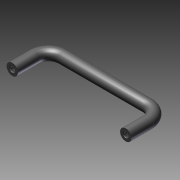
# Autodesk Inventor part: UWANGF_pull100-5
Saved by Autodesk Inventor 2015 SP1 (Build 190203100, 203)
## iProperties
Category: Hardware
Company: MISUMI
Created: 2015-01-28
Part Number: UWANGF_pull100-5
Catalog Web Link: http://us.misumi-ec.com/vona2/detail/110302025920/
Description: UWANGF, UWANSGF_pull-Pulls with Plates - Pull
Vendor: MISUMI
Document SubType Name: Modeling
Designer: psAdmin
Manufacturer: MISUMI
Mass: 11.5881 g
Surface Area: 53.4638 cm^2
Volume: 11.5881 cm^3
Density: 1 g/cm^3
Material: Generic
Appearance: PSOLRGB-192-192-192
Stock Number: UWANGF-100-5
PSOL_IDENT_0: {\\10.0.0.236\data_v8\23d-libs\misumi\metric\39_accessories_for_al_extrusions\uwangf_pull.prj},196 {
PSOL_IDENT_1: VTYP=3D},{NB=UWANGF_pull100-5},{LINA=UWANGF_pull100-5},{NN=UWANGF, UWANSGF_pull},{DATE=17.11.2014 05
PSOL_IDENT_2: :31:37},{GEOMDATE=14.09.2009 00:00:00},{VERSION=},{LINEID=20},{LINESUBID=-1},{WBVAR=MATMB,AF}  {NB=U
PSOL_IDENT_3: WANGF_pull100-5},{LINA=UWANGF_pull100-5},{KT=DUMMY},{PN=UWANGF_pull100-5},{TYPE=UWANGF_pull},{MATMB=
PSOL_IDENT_4: },{STMB=Chrome Plating},{MATP=Zinc Die Cast},{STP=Electrostatic Coating (Siliver)},{MATB=316 Stainle
PSOL_IDENT_5: ss Steel or Equivalent},{MATN=304 Stainless Steel or Equivalent},{MATT=304 Stainless Steel equivalen
PSOL_IDENT_6: t},{L=100},{AF=5},{AF1=5},{P=124},{L1=138},{ND=5},{NC=10.5},{LOAD=2000},{BOLT=SHFBS},{BOLTQ=4},{NUT=
PSOL_IDENT_7: HNTTSN},{NUTQ=2}
SUPPLIER: MISUMI
ARTICLENO: UWANGF_pull100-5
BOMINFO: UWANGF_pull100-5
CREATOR: CADENAS GmbH
Title: Handle
Author: Misumi
Autodesk Inventor part; units mm, degrees
sketch "Sketch_1" plane through (0, 0, 0) normal (0, 1, 0) x (-1, 0, 0)
  circle A0 centre (50, 0) radius 5
  constraints: 1 centre point
extrude "Extrusion1" add sketch "Sketch_1" along normal blind 19
sketch "Sketch_2" plane through (0, 19, 0) normal (0, 1, 0) x (1, 0, 0)
  line L0 (-37, 5) -> (-37, -5)
  circle A0 centre (-50, 0) radius 5
  constraints: 2 end point, 1 centre point
revolve "Revolution1" add sketch "Sketch_2" angle 90 about axis through (-37, 19, -5) along (0, 0, -1)
sketch "Sketch_3" plane through (-37, 0, 0) normal (1, 0, 0) x (0, 0, -1)
  circle A0 centre (0, 32) radius 5
  constraints: 1 centre point
extrude "Extrusion2" add sketch "Sketch_3" along normal blind 74
sketch "Sketch_4" plane through (0, 19, 0) normal (0, 1, 0) x (1, 0, 0)
  line L0 (37, -5) -> (37, 5)
  circle A0 centre (50, 0) radius 5
  constraints: 2 end point, 1 centre point
revolve "Revolution2" add sketch "Sketch_4" angle 90 about axis through (37, 19, 5) along (0, 0, 1)
sketch "Sketch_5" plane through (0, 0, 0) normal (0, 1, 0) x (-1, 0, 0)
  circle A0 centre (-50, 0) radius 5
  constraints: 1 centre point
extrude "Extrusion3" add sketch "Sketch_5" along normal blind 19
sketch "Sketch_6" plane through (0, 0, 0) normal (0, 0, 1) x (1, 0, 0)
  line L0 (-50, 0) -> (-50, 16.1934)
  line L1 (-50, 16.1934) -> (-47.933, 15)
  line L2 (-47.933, 15) -> (-47.933, 0.433)
  line L3 (-47.933, 0.433) -> (-47.5, 0)
  line L4 (-47.5, 0) -> (-50, 0)
  line L5 (-50, 0) -> (-50, 16.1934)
  constraints: 12 end point
revolve "Revolution3" cut sketch "Sketch_6" angle 360 about axis through (-50, 0, 0) along (0, -1, 0)
thread "Thread1" size "M5x0.8" class "6H" standard "ISO Metric profile" length 13 offset 2
sketch "Sketch_7" plane through (0, 0, 0) normal (0, 0, 1) x (1, 0, 0)
  line L0 (50, 0) -> (50, 16.1934)
  line L1 (50, 16.1934) -> (52.067, 15)
  line L2 (52.067, 15) -> (52.067, 0.433)
  line L3 (52.067, 0.433) -> (52.5, 0)
  line L4 (52.5, 0) -> (50, 0)
  line L5 (50, 0) -> (50, 16.1934)
  constraints: 12 end point
revolve "Revolution4" cut sketch "Sketch_7" angle 360 about axis through (50, 0, 0) along (0, -1, 0)
thread "Thread2" size "M5x0.8" class "6H" standard "ISO Metric profile" length 13 offset 2
ref_plane "bolt1_XY" through (-50, 0, 0) normal (0, 1, 0) x (1, 0, 0)
ref_plane "bolt1_YZ" through (-50, 0, 0) normal (1, 0, 0) x (0, 0, -1)
ref_plane "bolt1_ZX" through (-50, 0, 0) normal (0, 0, -1) x (0, 1, 0)
ref_plane "bolt2_XY" through (50, 0, 0) normal (0, 1, 0) x (1, 0, 0)
ref_plane "bolt2_YZ" through (50, 0, 0) normal (1, 0, 0) x (0, 0, -1)
ref_plane "bolt2_ZX" through (50, 0, 0) normal (0, 0, -1) x (0, 1, 0)
body "Solid1"
